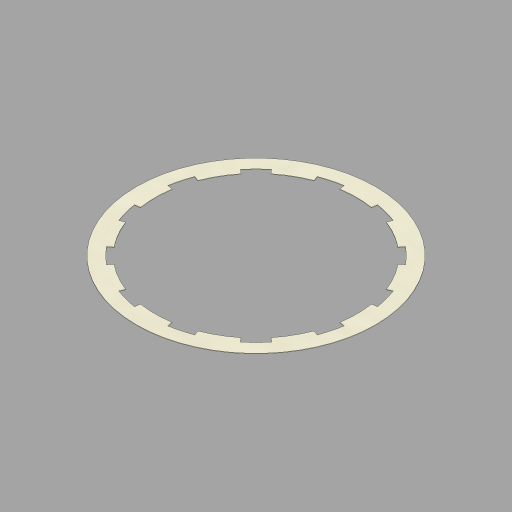
# Autodesk Inventor part: TorsionOscillator-IsolationRing
Saved by Autodesk Inventor 2024.2 (Build 282272000, 272)
## iProperties
Created: 2023-08-21
Part Number: TorsionOscillator-IsolationRing
Material: Paper
Document SubType Name: Modeling
Designer: schanen
Density: 0.93 g/cm^3
Appearance: Cardboard - Chipboard
Author: schanen
Autodesk Inventor part; units mm, degrees
ref_plane "YZ Plane" through (0, 0, 0) normal (1, 0, 0) x (0, 1, 0)
ref_plane "XZ Plane" through (0, 0, 0) normal (0, 1, 0) x (-1, 0, 0)
ref_plane "XY Plane" through (0, 0, 0) normal (0, 0, 1) x (1, 0, 0)
sketch "Sketch1" plane through (0, 0, 0) normal (0, 0, 1) x (1, 0, 0)
  line L0 (-20, 0) -> (-22.5, 0)
  line L1 (-22.5, 0) -> (-22.5, 0.1)
  line L2 (-22.5, 0.1) -> (-20, 0.1)
  line L3 (-20, 0.1) -> (-20, 0)
  line L4 (0, -0.02) -> (0, 0.12) projected
  point P0 (0, 0)
  dimension "d0" = 20
  dimension "d1" = 22.5
  dimension "d2" = 0.1
  constraints: 8 end point, 2 parallel, 1 horizontal, 1 perpendicular
  measures "d0" distance of point (0, 0) L0.start
  measures "d1" distance of point (0, 0) L0.end
  measures "d2" distance of L0.end L1.end
revolve "Revolution1" add sketch "Sketch1" angle 360 about axis through (0, -10, 0) along (0, 1, 0)
sketch "Sketch2" plane through (0, 0.1, 0) normal (0, 1, 0) x (1, 0, 0)
  circle A0 centre (0, 0) radius 19 construction
  line L0 (0, 0) -> (-19.7538, 3.1287)
  line L1 (0, 0) -> (-19.7538, -3.1287)
  circle A1 centre (0, 0) radius 20 projected
  circle A2 centre (0, 0) radius 20 projected
  arc A3 (-18.7661, 2.9723) -> (-18.7661, -2.9723) centre (0, 0) ccw
  arc A4 (-19.7538, 3.1287) -> (-19.7538, -3.1287) centre (0, 0) ccw
  point P0 (-19.7538, 3.1287)
  dimension "d4" = 38
  dimension "d5" = 18
  constraints: 7 point on circle, 4 end point, 3 centre point, 3 coincident, 2 point on line, 1 vertical alignment, 2 other
  measures "d4" diameter of A0
  measures "d5" angle of L1 L0
extrude "Extrusion1" add sketch "Sketch2" against normal up to surface (0.1 mm away) contours A3 L1 A1 L0
pattern_circular "Circular Pattern1" count 12 over 360 about axis through (0, 0.05, 0) along (0, 1, 0) of "Extrusion1"
body "Solid1"
